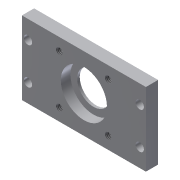
# Autodesk Inventor part: Module Top Plate
Saved by Autodesk Inventor 2014 SP1 (Build 180222100, 222)
## iProperties
Created: 2014-05-04
Part Number: Module Top Plate
Material: Aluminum 6061
Document SubType Name: Modeling
Designer: Rauhul Varma
Density: 2.71 g/cm^3
Appearance: Aluminum - Flat
Mass: 36.7057 g
Surface Area: 66.406 cm^2
Volume: 13.5445 cm^3
Author: Rauhul Varma
Autodesk Inventor part; units mm, degrees
ref_plane "YZ Plane" through (0, 0, 0) normal (1, 0, 0) x (0, 1, 0)
ref_plane "XZ Plane" through (0, 0, 0) normal (0, 1, 0) x (-1, 0, 0)
ref_plane "XY Plane" through (0, 0, 0) normal (0, 0, 1) x (1, 0, 0)
sketch "Sketch1" plane through (0, 0, 0) normal (0, 0, 1) x (1, 0, 0)
  line L0 (-32.2263, -19.05) -> (32.2263, -19.05)
  line L1 (32.2263, -19.05) -> (32.2263, 19.05)
  line L2 (32.2263, 19.05) -> (-32.2263, 19.05)
  line L3 (-32.2263, 19.05) -> (-32.2263, -19.05)
  line L4 (-32.2263, -19.05) -> (32.2263, 19.05) construction
  line L5 (32.2263, -19.05) -> (-32.2263, 19.05) construction
  line L6 (-25.8762, 19.05) -> (-25.8762, -19.05) construction
  line L7 (25.8762, 19.05) -> (25.8762, -19.05) construction
  line L8 (-29.0512, 19.05) -> (-29.0512, -19.05) construction
  line L9 (29.0512, 19.05) -> (29.0512, -19.05) construction
  line L10 (-32.2263, 0) -> (32.2263, 0) construction
  circle A0 centre (0, 0) radius 12
  circle A1 centre (0, 0) radius 8.5
  line L11 (-15.875, -15.875) -> (15.875, -15.875) construction
  line L12 (15.875, -15.875) -> (15.875, 15.875) construction
  line L13 (15.875, 15.875) -> (-15.875, 15.875) construction
  line L14 (-15.875, 15.875) -> (-15.875, -15.875) construction
  line L15 (-15.875, -15.875) -> (15.875, 15.875) construction
  line L16 (15.875, -15.875) -> (-15.875, 15.875) construction
  circle A2 centre (-12.7, 12.7) radius 3.175 construction
  line L17 (12.7, -12.7) -> (-12.7, -12.7) construction
  line L18 (-12.7, -12.7) -> (-12.7, 12.7) construction
  line L19 (-12.7, 12.7) -> (12.7, 12.7) construction
  line L20 (12.7, 12.7) -> (12.7, -12.7) construction
  line L21 (12.7, -12.7) -> (-12.7, 12.7) construction
  line L22 (-12.7, -12.7) -> (12.7, 12.7) construction
  point P0 (-29.0513, 9.525)
  point P1 (-29.0513, -9.525)
  point P2 (29.0512, -9.525)
  point P3 (29.0512, 9.525)
  dimension "d0" = 64.4525
  dimension "d1" = 38.1
  dimension "d2" = 6.35
  dimension "d3" = 6.35
  dimension "d4" = 9.525
  dimension "d5" = 9.525
  dimension "d6" = 24
  dimension "d18" = 17
  dimension "d19" = 31.75
  dimension "d20" = 31.75
  dimension "d21" = 6.35
  constraints: 46 end point, 13 point on line, 8 midpoint, 8 parallel, 6 coincident, 5 perpendicular, 3 centre point, 3 horizontal, 2 symmetric about line, 1 tangent, 2 other
  measures "d0" distance of L2.end L1.end
  measures "d1" distance of L1.end L0.end
  measures "d2" distance of L2.end L6.start
  measures "d3" distance of L1.end L7.start
  measures "d4" distance from line of L10 point (-29.051, -9.525)
  measures "d5" distance from line of L10 point (29.051, -9.525)
  measures "d6" diameter of A0
  measures "d18" diameter of A1
  measures "d19" distance of L13.end L12.end
  measures "d20" distance of L12.end L11.end
  measures "d21" diameter of A2
extrude "Extrusion1" add sketch "Sketch1" against normal blind 6.35 contours L3 L2 L1 L0 | A0
hole "Hole1" at (-29.0513, 9.525, 0) at (-29.0513, -9.525, 0) at (29.0512, -9.525, 0) at (29.0512, 9.525, 0) direction (0, 0, -1) diameter 4.318 end through all clearance for "Flat Head Machine Screw (82)" size "#8" standard "Ansi Unified Screw Threads"
extrude "Extrusion2" cut sketch "Sketch1" against normal blind 5 contours A0 | A1
hole "Hole2" at (-12.7, 12.7, 0) at (-12.7, -12.7, 0) at (12.7, -12.7, 0) at (12.7, 12.7, 0) direction (0, 0, -1) diameter 3.302 end through all thread size "8-32 UNC" class "2B" standard "ANSI Unified Screw Threads"
equation "\"d5\" = d4"
body "Solid1"
